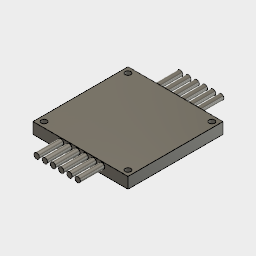
Spedix PDB v1 (Autodesk Fusion 360 design; units mm, degrees)
Autodesk Fusion 360 part; units mm, degrees
sketch "Sketch1" plane through (0, 0, 0) normal (0, 1, 0) x (1, 0, 0)
  line L0 (25.5, -25.5) -> (-25.5, -25.5)
  line L1 (-25.5, -25.5) -> (-25.5, 25.5)
  line L2 (-25.5, 25.5) -> (25.5, 25.5)
  line L3 (25.5, 25.5) -> (25.5, -25.5)
  line L4 (25.5, -25.5) -> (-25.5, 25.5) construction
  line L5 (-25.5, -25.5) -> (25.5, 25.5) construction
  circle A0 centre (-22.5, 22.5) radius 1.5
  circle A1 centre (22.5, 22.5) radius 1.5
  circle A2 centre (22.5, -22.5) radius 1.5
  circle A3 centre (-22.5, -22.5) radius 1.5
  dimension "d1" = 51
  dimension "d2" = 51
  dimension "d5" = 3
  dimension "d6" = 45
  measures "d1" distance of L1.end L2.end
  measures "d2" distance of L0.end L1.end
  measures "d5" diameter of A0
  measures "d6" distance of A0.centre A1.centre
extrude "Extrude1" add sketch "Sketch1" along normal blind 6
sketch "Sketch2" plane through (0, 0, 25.5) normal (0, 0, 1) x (1, 0, 0)
  line L0 (-25.5, 0) -> (25.5, 0)
  line L1 (25.5, 0) -> (25.5, 6)
  line L2 (25.5, 6) -> (-25.5, 6)
  line L3 (-25.5, 6) -> (-25.5, 0)
  circle A0 centre (-10.5, 4) radius 1.5
  circle A1 centre (-6.1, 4) radius 1.5
  circle A2 centre (-1.7, 4) radius 1.5
  circle A3 centre (2.7, 4) radius 1.5
  circle A4 centre (7.1, 4) radius 1.5
  circle A5 centre (11.5, 4) radius 1.5
  dimension "d7" = 3
  dimension "d8" = 2
  dimension "d9" = 15
  dimension "d12" = -22
  dimension "d13" = 0
  measures "d7" diameter of A0
  measures "d8" distance of L2 A0.centre
  measures "d9" distance of L3 A0.centre
extrude "Extrude2" add sketch "Sketch2" along normal blind 13 contours A0 | A1 | A2 | A3 | A4 | A5
mirror "Mirror1" about plane through (0, 0, 0) normal (0, 0, 1) of "Extrude2"
